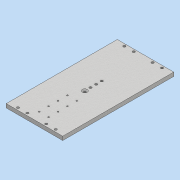
# Autodesk Inventor part: Wspornik pionowy osi Z
Saved by Autodesk Inventor 2018 (Build 220112000, 112)
## iProperties
Created: 2019-01-27
Part Number: Wspornik pionowy osi Z
Material: Ogólny
Document SubType Name: Modeling
Designer: Dawid
Density: 1 g/cm^3
Appearance: Aluminium odlewane
Author: Dawid
Autodesk Inventor part; units mm, degrees
ref_plane "YZ Plane" through (0, 0, 0) normal (1, 0, 0) x (0, 1, 0)
ref_plane "XZ Plane" through (0, 0, 0) normal (0, 1, 0) x (-1, 0, 0)
ref_plane "XY Plane" through (0, 0, 0) normal (0, 0, 1) x (1, 0, 0)
sketch "Szkic1" plane through (0, 0, 0) normal (0, 0, 1) x (1, 0, 0)
  line L0 (-50, -65) -> (50, -65)
  line L1 (50, -65) -> (50, 65)
  line L2 (50, 65) -> (-50, 65)
  line L3 (-50, 65) -> (-50, -65)
  line L4 (-50, -65) -> (50, 65) construction
  line L5 (50, -65) -> (-50, 65) construction
  point P0 (0, 0)
  dimension "d0" = 100
  dimension "d1" = 130
  constraints: 12 end point, 2 midpoint, 2 parallel, 1 horizontal, 1 perpendicular
  measures "d0" distance of L2.end L1.end
  measures "d1" distance of L1.end L0.end
extrude "Wyciągnięcie proste1" add sketch "Szkic1" along normal blind 8
sketch "Szkic7" plane through (-50, 65, 0) normal (0, 1, 0) x (1, 0, 0)
  line L0 (100, 0) -> (0, 0) projected
  line L1 (0, 0) -> (0, -8) projected
  line L2 (100, -8) -> (0, -8) projected
  line L3 (100, 0) -> (100, -8) projected
  point P0 (50, 0)
extrude "Wyciągnięcie proste6" add sketch "Szkic7" along normal blind 45
sketch "Szkic9" plane through (0, 0, 0) normal (0, 0, -1) x (-1, 0, 0)
  circle A0 centre (-10, -5) radius 1.5
  circle A1 centre (-10, 15) radius 1.5
  circle A2 centre (10, -5) radius 1.5
  circle A3 centre (10, 15) radius 1.5
  circle A4 centre (-10, -45) radius 1.5
  circle A5 centre (-10, -25) radius 1.5
  circle A6 centre (10, -45) radius 1.5
  circle A7 centre (10, -25) radius 1.5
  line L0 (50, -65) -> (-50, -65) projected
  line L1 (50, -65) -> (50, 110) projected
  line L2 (-50, 110) -> (50, 110) projected
  line L3 (-50, -65) -> (-50, 110) projected
  circle A8 centre (-10, -45) radius 1.5
  circle A9 centre (-10, -55) radius 1.5 projected
  line L4 (-10, -55) -> (-10, -45)
  point P0 (0, 10)
  dimension "d119" = 10
  constraints: 17 centre point, 2 end point, 1 vertical
  measures "d119" distance of L4.start L4.end
hole "Otwór2" at (10, 15, 0) at (-10, 15, 0) at (-10, -5, 0) at (10, -5, 0) at (10, -25, 0) at (-10, -25, 0) at (-10, -45, 0) at (10, -45, 0) direction (0, 0, 1) diameter 3 end through all countersink diameter 7 countersink angle 90
sketch "Szkic10" plane through (50, -65, 8) normal (1, 0, 0) x (0, 0, -1)
  line L0 (8, 0) -> (8, 175) projected
  line L1 (0, 175) -> (8, 175) projected
  line L2 (0, 0) -> (0, 175) projected
  line L3 (8, 0) -> (0, 0) projected
  point P0 (8, 65)
sketch "Szkic11" plane through (-50, -65, 0) normal (-1, 0, 0) x (0, 0, 1)
  line L0 (0, 0) -> (0, 175) projected
  line L1 (0, 0) -> (8, 0) projected
  line L2 (8, 0) -> (8, 175) projected
  line L3 (0, 175) -> (8, 175) projected
  point P0 (0, 65)
extrude "Wyciągnięcie proste8" add sketch "Szkic11" along normal blind 10
extrude "Wyciągnięcie proste9" add sketch "Szkic10" along normal blind 10
sketch "Szkic14" plane through (0, 0, 8) normal (0, 0, 1) x (1, 0, 0)
  line L0 (60, -75) -> (-60, -75) projected
  line L1 (-60, -65) -> (-60, 110) projected
  line L2 (60, 110) -> (60, -65) projected
  line L3 (-60, -65) -> (-60, -55)
  line L4 (-60, 110) -> (-60, -65) projected
  line L5 (-60, -55) -> (60, -55)
  line L6 (-60, -55) -> (-60, -60)
  line L7 (-60, -60) -> (60, -60)
  line L8 (-60, -65) -> (-40, -65)
  line L9 (-60, -75) -> (60, -75) projected
  line L10 (-40, -65) -> (-40, -55)
  line L11 (-40, -65) -> (-20, -65)
  line L12 (-20, -65) -> (-20, -55)
  line L13 (-20, -65) -> (20, -65)
  line L14 (20, -65) -> (20, -55)
  line L15 (20, -65) -> (40, -65)
  line L16 (40, -65) -> (40, -55)
  circle A0 centre (-40, -60) radius 2.5
  circle A1 centre (-20, -60) radius 2.5
  circle A2 centre (20, -60) radius 2.5
  circle A3 centre (40, -60) radius 2.5
  line L17 (-60, -65) -> (-60, -55)
  point P0 (0, 0)
  dimension "d84" = 20
  dimension "d85" = 5
  dimension "d87" = 20
  dimension "d89" = 20
  dimension "d90" = 5
  dimension "d91" = 5
  dimension "d92" = 5
  dimension "d93" = 5
  dimension "d105" = 20
  dimension "d120" = 10
  dimension "d121" = 20
  constraints: 26 end point, 6 perpendicular, 5 point on line, 4 centre point, 4 midpoint
  measures "d84" distance of L0.end L3.end
  measures "d85" distance of L3.end L6.end
  measures "d87" distance of L8.end L11.end
  measures "d89" distance of L13.end L15.end
  measures "d90" diameter of A0
  measures "d91" diameter of A1
  measures "d92" diameter of A2
  measures "d93" diameter of A3
  measures "d105" distance from line of L2 A3.centre
  measures "d120" distance of L17.start L17.end
  measures "d121" distance from line of L1 A0.centre
hole "Otwór5" at (-40, -60, 8) at (-20, -60, 8) at (20, -60, 8) at (40, -60, 8) direction (0, 0, -1) diameter 5 end through all
sketch "Szkic16" plane through (-50, 110, 0) normal (0, 1, 0) x (1, 0, 0)
  line L0 (-10, 0) -> (110, 0) projected
  line L1 (-10, -8) -> (-10, 0) projected
  line L2 (110, -8) -> (-10, -8) projected
  line L3 (110, 0) -> (110, -8) projected
  point P0 (50, 0)
extrude "Wyciągnięcie proste12" add sketch "Szkic16" along normal blind 61
sketch "Szkic17" plane through (0, 0, 0) normal (0, 0, -1) x (-1, 0, 0)
  line L0 (60, 161) -> (-60, 161)
  line L1 (-60, 346) -> (-60, 161)
  line L2 (60, 346) -> (60, 161)
  line L3 (-60, 161) -> (-60, 171)
  line L4 (-60, 346) -> (-60, 161)
  line L5 (-60, 171) -> (60, 171)
  line L6 (-60, 171) -> (-60, 166)
  line L7 (-60, 166) -> (60, 166)
  line L8 (-60, 161) -> (-40, 161)
  line L9 (-60, 161) -> (60, 161)
  line L10 (-40, 161) -> (-40, 171)
  line L11 (-40, 161) -> (-20, 161)
  line L12 (-20, 161) -> (-20, 171)
  line L13 (-20, 161) -> (20, 161)
  line L14 (20, 161) -> (20, 171)
  line L15 (20, 161) -> (40, 161)
  line L16 (40, 161) -> (40, 171)
  circle A0 centre (-40, 166) radius 2.5
  circle A1 centre (-20, 166) radius 2.5
  circle A2 centre (20, 166) radius 2.5
  circle A3 centre (40, 166) radius 2.5
  line L17 (-60, 171) -> (60, 171) projected
  point P0 (0, 0)
  point P1 (0, 236)
  dimension "d106" = 10
  dimension "d107" = 5
  dimension "d108" = 20
  dimension "d109" = 20
  dimension "d110" = 20
  dimension "d111" = 5
  dimension "d112" = 5
  dimension "d113" = 5
  dimension "d114" = 5
  dimension "d115" = 20
  constraints: 34 end point, 12 point on line, 6 perpendicular, 4 centre point, 4 midpoint
  measures "d106" distance of L0.end L3.end
  measures "d107" distance of L3.end L6.end
  measures "d108" distance of L0.end L8.end
  measures "d109" distance of L8.end L11.end
  measures "d110" distance of L13.end L15.end
  measures "d111" diameter of A0
  measures "d112" diameter of A1
  measures "d113" diameter of A2
  measures "d114" diameter of A3
  measures "d115" distance from line of L2 A3.centre
extrude "Wyciągnięcie proste13" cut sketch "Szkic17" against normal up to next contours A3 L7 L16 | L16 L7 A3 | L7 L16 A3 | A2 L7 L14 | L14 L7 A2 | L7 A3 L16 | A1 L7 L12 | L12 L7 A1 | L14 A2 L7 | L7 A2 L14 | A0 L7 L10 | L10 L7 A0 | L12 A1 L7 | L7 A1 L12 | L10 A0 L7 | L7 A0 L10
sketch "Szkic18" plane through (0, 0, 8) normal (0, 0, 1) x (1, 0, 0)
  line L0 (10, 30) -> (10, 90)
  line L1 (10, 90) -> (-10, 90)
  line L2 (-10, 90) -> (-10, 30)
  line L3 (10, 30) -> (-10, 30)
  line L4 (-10, 30) -> (-10, 90)
  line L5 (-10, 30) -> (0, 30)
  line L6 (0, 30) -> (0, 90)
  line L7 (10, 90) -> (-10, 90)
  line L8 (0, 30) -> (0, 42)
  line L9 (0, 42) -> (0, 54)
  line L10 (0, 54) -> (0, 66)
  line L11 (0, 66) -> (0, 78)
  circle A0 centre (0, 42) radius 2.5
  circle A1 centre (0, 54) radius 2.5
  circle A2 centre (0, 66) radius 2.5
  circle A3 centre (0, 78) radius 2.5
  line L12 (-60, 171) -> (60, 171) projected
  line L13 (60, -65) -> (60, 171) projected
  line L14 (60, -65) -> (60, 171) projected
  line L15 (60, 171) -> (60, 90)
  line L16 (60, 90) -> (0, 90)
  line L17 (-60, -65) -> (-60, 171) projected
  line L18 (0, 171) -> (0, -65)
  line L19 (60, -65) -> (-60, -65) projected
  point P0 (0, 0)
  point P1 (13, 60)
  dimension "d122" = 10
  dimension "d123" = 12
  dimension "d124" = 12
  dimension "d125" = 12
  dimension "d126" = 12
  dimension "d127" = 5
  dimension "d128" = 5
  dimension "d129" = 5
  dimension "d130" = 5
  dimension "d131" = 81
  constraints: 30 end point, 6 point on line, 4 centre point, 4 coincident, 4 midpoint, 1 perpendicular
  measures "d122" distance of L2.end L5.end
  measures "d123" distance of L5.end L8.end
  measures "d124" distance of L8.end L9.end
  measures "d125" distance of L9.end L10.end
  measures "d126" distance of L10.end L11.end
  measures "d127" diameter of A0
  measures "d128" diameter of A1
  measures "d129" diameter of A2
  measures "d130" diameter of A3
  measures "d131" distance of L12.end L15.end
extrude "Wyciągnięcie proste14" cut sketch "Szkic18" against normal up to next contours A0 L6 | L6 A0 | A3 L6 | L6 A3 | A1 L6 | L6 A1 | A2 L6 | L6 A2
hole "Otwór6" at (0, 78, 0) direction (0, 0, 1) diameter 5 end through all countersink diameter 10.5 countersink angle 90
hole "Otwór7" at (0, 66, 0) direction (0, 0, 1) diameter 5 end through all countersink diameter 10.5 countersink angle 90
hole "Otwór8" at (0, 42, 8) direction (0, 0, -1) diameter 5 end through all countersink diameter 10.5 countersink angle 90
hole "Otwór9" at (0, 54, 0) direction (0, 0, 1) diameter 5 end through all countersink diameter 10.5 countersink angle 90
hole "Otwór10" at (0, 42, 0) direction (0, 0, 1) diameter 5 end through all countersink diameter 10.5 countersink angle 90
